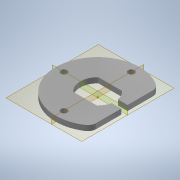
# Autodesk Inventor part: PaDC motor connectie part 2
Saved by Autodesk Inventor 2021 (Build 250183000, 183)
## iProperties
Manager: PJ / DCS
Company: Emmaüs Bovenbouw Aalter
Created: 2021-01-09
Part Number: PaDC motor connectie part 2
Material: S235
Catalog Web Link: http://emmausbovenbouw.op-weg.be/
Vendor: Emmaüsinstituut Bovenbouw Aalter
Document SubType Name: Modeling
Designer: Antho
Engineer: Declercq St.
Manufacturer: Standard
Standards Organization: Custom
Density: 7.86 g/cm^3
Appearance: Steel
Title: Algemene titel
Subject: Specifieke titel
Author: Antho
Keywords: Ruwe Ø xxxxx
Comments: Opmerking
Autodesk Inventor part; units mm, degrees
sketch "Sketch1" plane through (0, 0, 0) normal (0, 0, 1) x (1, 0, 0)
  line L0 (0, 3.811) -> (0, -3.811) construction
  line L1 (-7.7033, 0) -> (7.7033, 0) construction
  circle A0 centre (0, 0) radius 20
  dimension "d0" = 40
  constraints: 4 end point, 2 coincident, 2 midpoint, 1 centre point, 1 horizontal, 1 vertical
  measures "d0" diameter of A0
extrude "Extrusion1" add sketch "Sketch1" along normal blind 2.5
sketch "Sketch2" plane through (0, 0, 2.5) normal (0, 0, 1) x (1, 0, 0)
  line L0 (0, 0) -> (0, -16)
  line L1 (0, 0) -> (16, 0) construction
  line L2 (0, 0) -> (-16, 0)
  line L3 (0, 0) -> (16, 0) construction
  line L4 (0, 0) -> (0, 16)
  line L5 (0, 0) -> (16, 0) construction
  line L6 (0, 0) -> (16, 0)
  dimension "d18" = 16
  dimension "d19" = 90
  dimension "d20" = 16
  dimension "d21" = 180
  dimension "d22" = 16
  dimension "d23" = 90
  dimension "d24" = 16
  dimension "d43" = 0
  constraints: 14 end point, 4 coincident, 3 equal length, 3 horizontal
  measures "d18" distance of L0.start L0.end
  measures "d19" angle of L0 L1
  measures "d20" distance of L0.start L2.end
  measures "d21" angle of L3 L2
  measures "d22" distance of L0.start L4.end
  measures "d23" angle of L5 L4
  measures "d24" distance of L0.start L6.end
  measures "d43" distance between parallel lines of L1 L6
hole "Hole1" at (-16, 0, 2.5) at (0, 16, 2.5) at (16, 0, 2.5) at (0, -16, 2.5) direction (0, 0, -1) diameter 3 depth 2.5
sketch "Sketch3" plane through (0, 0, 2.5) normal (0, 0, 1) x (1, 0, 0)
  line L0 (-6, -5.6624) -> (6, 5.6624) construction
  line L1 (6, -5.6624) -> (-6, 5.6624) construction
  line L2 (-5.6624, -6) -> (5.6624, -6)
  line L3 (5.6624, -6) -> (5.6624, 6)
  line L4 (5.6624, 6) -> (-5.6624, 6)
  line L5 (-5.6624, 6) -> (-5.6624, -6)
  line L6 (-5.6624, -6) -> (5.6624, 6) construction
  line L7 (5.6624, -6) -> (-5.6624, 6) construction
  arc A0 (6, 5.6624) -> (5.6624, 6) centre (0, 0) ccw
  arc A1 (-5.6624, 6) -> (-6, 5.6624) centre (0, 0) ccw
  arc A2 (-6, -5.6624) -> (-5.6624, -6) centre (0, 0) ccw
  arc A3 (5.6624, -6) -> (6, -5.6624) centre (0, 0) ccw
  arc A4 (-5.6624, 6) -> (-5.6624, -6) centre (0, 0) ccw
  arc A5 (5.6624, -6) -> (5.6624, 6) centre (0, 0) ccw
  arc A6 (-5.6624, 6) -> (-5.6624, -6) centre (0, 0) ccw
  arc A7 (5.6624, -6) -> (5.6624, 6) centre (0, 0) ccw
  point P0 (6, -5.6624)
  point P1 (-6, 5.6624)
  dimension "d52" = 12
  constraints: 16 end point, 16 point on circle, 8 centre point, 4 midpoint, 2 coincident, 2 parallel, 1 horizontal, 1 perpendicular
  measures "d52" distance of L3.end L2.end
extrude "Extrusion2" cut sketch "Sketch3" against normal blind 2.5
sketch "Sketch5" plane through (0, 0, 2.5) normal (0, 0, 1) x (1, 0, 0)
  circle A0 centre (0, 0) radius 12.7095
  circle A1 centre (0, 16) radius 1.5 projected
  line L0 (0, 0) -> (0, 16)
  line L1 (12.7095, 0) -> (12.7095, 20)
  line L2 (12.7095, 20) -> (22.7095, 20)
  line L3 (22.7095, 20) -> (22.7095, -20)
  line L4 (22.7095, -20) -> (12.7095, -20)
  line L5 (12.7095, -20) -> (12.7095, 20)
  dimension "d37" = 25.419
  dimension "d44" = 20
  dimension "d45" = 10
  dimension "d46" = 40
  constraints: 12 end point, 3 parallel, 1 coincident, 1 horizontal, 1 horizontal alignment, 1 perpendicular, 1 vertical, 2 other
  measures "d44" distance of L1.start L1.end
  measures "d45" distance of L3.end L4.end
  measures "d46" distance of L2.end L3.end
extrude "Extrusion4" cut sketch "Sketch5" against normal blind 10 contours L1 L2 L3 L4 L5
fillet "Fillet1" radius 4 2 edges at (12.7095, -15.4424, 1.25) (12.7095, 15.4424, 1.25)
sketch "Sketch6" plane through (0, 0, 2.5) normal (0, 0, 1) x (1, 0, 0)
  line L0 (6, 5.6624) -> (6, -5.6624) projected
  line L1 (6, 0) -> (12.7095, 0)
  line L2 (12.7095, 13.4218) -> (12.7095, -13.4218) projected
  line L3 (9.3548, 0) -> (9.3548, -1)
  line L4 (6, -1.5) -> (12.7095, -1.5)
  line L5 (12.7095, -1.5) -> (12.7095, 1.5)
  line L6 (12.7095, 1.5) -> (6, 1.5)
  line L7 (6, 1.5) -> (6, -1.5)
  line L8 (6, -1.5) -> (12.7095, 1.5) construction
  line L9 (12.7095, -1.5) -> (6, 1.5) construction
  point P0 (0, 0)
  dimension "d47" = 1
  dimension "d48" = 3
  constraints: 16 end point, 5 midpoint, 2 parallel, 1 horizontal, 1 perpendicular, 1 point on line, 1 vertical
  measures "d47" distance of L3.start L3.end
  measures "d48" distance of L5.end L4.end
extrude "Extrusion5" cut sketch "Sketch6" against normal blind 10
body "Solid1"
